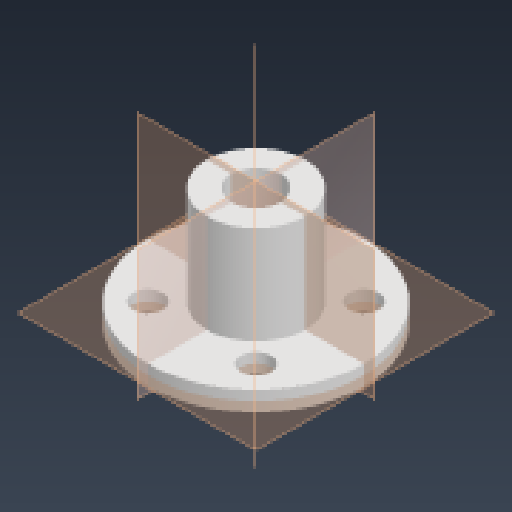
# Autodesk Inventor part: Фланцевая_муфта
Saved by Autodesk Inventor 2023.2 (Build 272271030, 271C)
## iProperties
Created: 2025-12-24
Part Number: Фланцевая_муфта
Material: Типовые
Document SubType Name: Modeling
Designer: Олег Коноваленко
Density: 1 g/cm^3
Appearance: По умолчанию
Author: Олег Коноваленко
Autodesk Inventor part; units mm, degrees
sketch "Эскиз1" plane through (0, 0, 0) normal (0, 1, 0) x (-1, 0, 0)
  circle A0 centre (0, 0) radius 11
  circle A1 centre (5.5, -5.5) radius 1.5
  circle A2 centre (5.5, 5.5) radius 1.5
  circle A3 centre (-5.5, 5.5) radius 1.5
  circle A4 centre (-5.5, -5.5) radius 1.5
  line L0 (5.5, -5.5) -> (-5.5, -5.5) construction
  line L1 (-5.5, -5.5) -> (-5.5, 5.5) construction
  line L2 (-5.5, 5.5) -> (5.5, 5.5) construction
  line L3 (5.5, 5.5) -> (5.5, -5.5) construction
  line L4 (5.5, -5.5) -> (-5.5, 5.5) construction
  line L5 (-5.5, -5.5) -> (5.5, 5.5) construction
  circle A5 centre (0, 0) radius 2.5
  dimension "d0" = 22
  dimension "d1" = 3
  dimension "d2" = 11
  dimension "d5" = 5
  constraints: 12 end point, 6 centre point, 3 coincident, 3 equal radius, 2 horizontal, 2 vertical, 1 midpoint, 1 perpendicular
  measures "d0" diameter of A0
  measures "d1" diameter of A1
  measures "d2" distance of L0.start L0.end
  measures "d5" diameter of A5
extrude "Выдавливание1" add sketch "Эскиз1" along normal mid plane 2
sketch "Эскиз2" plane through (0, 1, 0) normal (0, 1, 0) x (1, 0, 0)
  circle A0 centre (0, 0) radius 5
  circle A1 centre (0, 0) radius 2.5 projected
  dimension "d6" = 10
  constraints: 1 centre point, 1 coincident
  measures "d6" diameter of A0
extrude "Выдавливание2" add sketch "Эскиз2" along normal blind 10
ref_plane "РабПлоскость1" through (0, 0, 0) normal (0.7071, 0, -0.7071) x (0, 1, 0)
